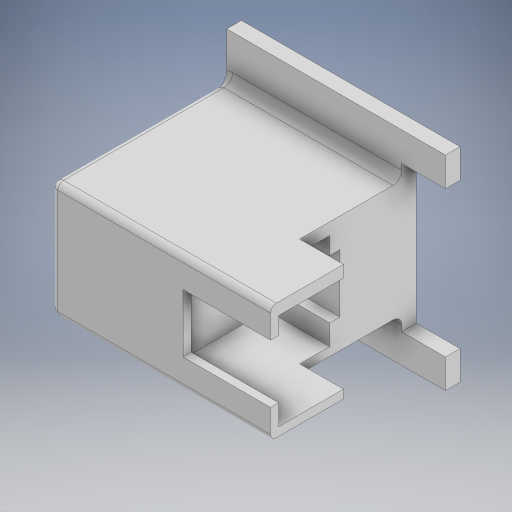
# Autodesk Inventor part: Base
Saved by Autodesk Inventor 2024 (Build 280153000, 153)
## iProperties
Created: 2023-08-21
Part Number: Base
Material: Generic
Document SubType Name: Modeling
Designer: arrusr01
Density: 1 g/cm^3
Appearance: Default
Author: arrusr01
Autodesk Inventor part; units mm, degrees
ref_plane "YZ Plane" through (0, 0, 0) normal (1, 0, 0) x (0, 1, 0)
ref_plane "XZ Plane" through (0, 0, 0) normal (0, 1, 0) x (-1, 0, 0)
ref_plane "XY Plane" through (0, 0, 0) normal (0, 0, 1) x (1, 0, 0)
sketch "Sketch1" plane through (0, 0, 0) normal (0, 0, 1) x (1, 0, 0)
  line L0 (-37.5, -35) -> (37.5, -35)
  line L1 (37.5, -35) -> (37.5, 35)
  line L2 (37.5, 35) -> (-37.5, 35)
  line L3 (-37.5, 35) -> (-37.5, -35)
  line L4 (-37.5, -35) -> (37.5, 35) construction
  line L5 (37.5, -35) -> (-37.5, 35) construction
  point P0 (0, 0)
  dimension "d0" = 70
  dimension "d1" = 75
  constraints: 12 end point, 2 midpoint, 2 parallel, 1 horizontal, 1 perpendicular
  measures "d0" distance of L2.end L0.start
  measures "d1" distance of L1.end L2.end
extrude "Extrusion1" add sketch "Sketch1" along normal blind 5
sketch "Sketch2" plane through (0, 0, 5) normal (0, 0, 1) x (1, 0, 0)
  line L0 (37.5, -35) -> (37.5, 35) projected
  line L1 (-37.5, 20) -> (37.5, 20)
  line L2 (37.5, 20) -> (37.5, -20)
  line L3 (37.5, -20) -> (-37.5, -20)
  line L4 (-37.5, -20) -> (-37.5, 20)
  line L5 (-37.5, 20) -> (37.5, -20) construction
  line L6 (37.5, 20) -> (-37.5, -20) construction
  point P0 (0, 0)
  dimension "d4" = 40
  constraints: 12 end point, 2 midpoint, 2 parallel, 1 horizontal, 1 perpendicular, 1 point on line
  measures "d4" distance of L3.end L1.start
extrude "Extrusion2" add sketch "Sketch2" along normal blind 60
sketch "Sketch4" plane through (0, 0, 65) normal (0, 0, 1) x (1, 0, 0)
  line L0 (37.5, -20) -> (37.5, 20) construction
  line L1 (37.5, 0) -> (7.5, 0)
  line L2 (7.5, 0) -> (7.5, 10)
  line L3 (7.5, 10) -> (37.5, 10)
  line L4 (37.5, 20) -> (37.5, -20) construction
  line L5 (7.5, 0) -> (7.5, -10)
  line L6 (7.5, -10) -> (37.5, -10)
  line L7 (37.5, 10) -> (37.5, -10)
  point P0 (0, 0)
  dimension "d14" = 10
  constraints: 14 end point, 4 symmetric about line, 1 collinear, 1 horizontal, 1 midpoint, 1 perpendicular, 1 vertical
  measures "d14" distance of L1.end L2.end
extrude "Extrusion4" cut sketch "Sketch4" against normal blind 36
sketch "Sketch5" plane through (37.5, -35, 0) normal (1, 0, 0) x (0, 0, -1)
  line L0 (-65, 25) -> (-65, 45) projected
  line L1 (-65, 34.4375) -> (-62.222, 34.4375)
  line L2 (-62.222, 34.4375) -> (-62.222, 17.9375)
  line L3 (-62.222, 17.9375) -> (-29.722, 17.9375)
  line L4 (-62.222, 34.4375) -> (-62.222, 50.9375)
  line L5 (-62.222, 50.9375) -> (-29.722, 50.9375)
  line L6 (-29.722, 17.9375) -> (-29.722, 50.9375)
  line L7 (-65, 25) -> (-29, 25) projected
  point P0 (0, 35)
  dimension "d17" = 16.5
  dimension "d18" = 32.5
  constraints: 12 end point, 3 perpendicular, 2 symmetric about line, 1 horizontal, 1 point on line
  measures "d17" distance of L1.end L2.end
  measures "d18" distance of L2.end L3.end
extrude "Extrusion5" cut sketch "Sketch5" against normal blind 36.5 contours L7 L6 L3 L2 | L2 L4 L5 L6 L7
sketch "Sketch6" plane through (37.5, -35, 0) normal (1, 0, 0) x (0, 0, -1)
  line L0 (-29.722, 25) -> (-29.722, 17.9375) projected
  line L1 (-29.722, 25) -> (-26.222, 25)
  line L2 (-26.222, 25) -> (-26.222, 45)
  line L3 (-26.222, 45) -> (-29.722, 45)
  line L4 (-29.722, 45) -> (-29.722, 25)
  point P0 (0, 35)
  dimension "d21" = 3.5
  constraints: 8 end point, 2 parallel, 1 horizontal, 1 perpendicular
  measures "d21" distance of L0.start L1.end
extrude "Extrusion6" cut sketch "Sketch6" against normal blind 30
sketch "Sketch8" plane through (0, 0, 0) normal (0, 0, -1) x (-1, 0, 0)
  line L0 (-37.5, 10) -> (-37.5, -10) projected
  line L1 (-37.5, 0) -> (-37.5, -25)
  line L2 (-37.5, -25) -> (-22.5, -25)
  line L3 (-22.5, -25) -> (-22.5, 0)
  line L4 (-22.5, 0) -> (-37.5, 0) construction
  line L5 (-37.5, 0) -> (-37.5, 25)
  line L6 (-37.5, 25) -> (-22.5, 25)
  line L7 (-22.5, 25) -> (-22.5, 0)
  point P0 (0, 0)
  dimension "d28" = 25
  dimension "d29" = 15
  constraints: 14 end point, 2 perpendicular, 2 symmetric about line, 2 vertical, 1 midpoint
  measures "d28" distance of L1.start L1.end
  measures "d29" distance of L1.end L2.end
extrude "Extrusion8" cut sketch "Sketch8" against normal blind 40
fillet "Fillet1" radius 2 5 edges at (0, -20, 65) (0, 20, 65) (-37.5, 0, 65) (-37.5, -20, 35) (-37.5, 20, 35)
fillet "Fillet2" radius 3 4 edges at (-36.9142, 19.4142, 5) (-6.5, 20, 5) (-36.9142, -19.4142, 5) (-6.5, -20, 5)
body "Solid1"
